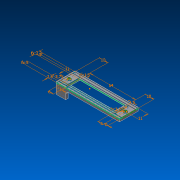
# Autodesk Inventor part: ethernet bracket
Saved by Autodesk Inventor 2015 (Build 190159000, 159)
## iProperties
Created: 2017-03-16
Part Number: ethernet bracket
Material: Generic
Document SubType Name: Modeling
Designer: ZigZagJoe
Density: 1 g/cm^3
Appearance: Default
Author: ZigZagJoe
Autodesk Inventor part; units mm, degrees
ref_plane "YZ Plane" through (0, 0, 0) normal (1, 0, 0) x (0, 1, 0)
ref_plane "XZ Plane" through (0, 0, 0) normal (0, 1, 0) x (-1, 0, 0)
ref_plane "XY Plane" through (0, 0, 0) normal (0, 0, 1) x (1, 0, 0)
sketch "Sketch1" plane through (0, 0, 0) normal (0, 0, 1) x (1, 0, 0)
  line L0 (-15.681, 3.6583) -> (38.319, 3.6583)
  line L1 (38.319, 3.6583) -> (38.319, -8.3417)
  line L2 (38.319, -8.3417) -> (-15.681, -8.3417)
  line L3 (-15.681, -8.3417) -> (-15.681, 3.6583)
  line L4 (48.319, 8.6583) -> (-25.681, 8.6583)
  line L5 (-25.681, 8.6583) -> (-25.681, -13.3417)
  line L6 (-25.681, -13.3417) -> (48.319, -13.3417)
  line L7 (48.319, -13.3417) -> (48.319, 8.6583)
  line L8 (-25.681, 5.8583) -> (48.319, 5.8583)
  line L9 (-25.681, -10.5417) -> (-25.681, -13.3417)
  line L10 (-25.681, -10.5417) -> (-14.681, -10.5417)
  line L11 (-14.681, -13.3417) -> (-25.681, -13.3417)
  line L12 (-25.681, -13.3417) -> (-25.681, -10.5417)
  line L13 (-14.681, -10.5417) -> (-14.681, -13.3417)
  line L14 (-14.681, -10.5417) -> (48.319, -10.5417)
  point P0 (0, 0)
  dimension "d0" = 54
  dimension "d1" = 12
  dimension "d4" = 5
  dimension "d5" = 5
  dimension "d7" = 2.2
  dimension "d62" = 10
  dimension "d65" = 10
  dimension "d66" = 0
  dimension "d69" = 1
  dimension "d70" = 2.8
  constraints: 31 end point, 6 point on line, 5 horizontal, 5 parallel, 2 perpendicular, 1 vertical
  measures "d0" distance of L1.end L2.end
  measures "d1" distance of L0.end L1.end
  measures "d4" distance between parallel lines of L4 L0
  measures "d5" distance between parallel lines of L2 L6
  measures "d7" distance between parallel lines of L8 L0
  measures "d62" distance between parallel lines of L3 L5
  measures "d65" distance between parallel lines of L7 L1
  measures "d66" distance of L6.end point (48.319, -13.342)
  measures "d69" distance between parallel lines of L13 L3
  measures "d70" distance between parallel lines of L11 L10
extrude "Face" add sketch "Sketch1" along normal blind 1
extrude "Walls" add sketch "Sketch1" against normal blind 3 contours L7 L8 L5 L4 | L7 L6 L13 L14 | L10 L13 L6 L5
extrude "Screw Support" add sketch "Sketch1" against normal blind 12 contours L10 L13 L6 L5
fillet "Fillet3" radius 0.5 1 edges at (11.319, 5.8583, 0)
sketch "Sketch2" plane through (-25.681, 5.8583, -3) normal (0, -1, 0) x (1, 0, 0)
  line L0 (56.5, 0.5) -> (53, 0.5)
  line L1 (53, 0.5) -> (53, 2)
  line L2 (53, 2) -> (56.5, 2)
  line L3 (56.5, 2) -> (56.5, 0.5)
  line L4 (21, 0.5) -> (17.5, 0.5)
  line L5 (17.5, 0.5) -> (17.5, 2)
  line L6 (17.5, 2) -> (21, 2)
  line L7 (21, 2) -> (21, 0.5)
  line L8 (74, 2.5) -> (74, 0) projected
  line L9 (0, 2.5) -> (0, 0) projected
  line L10 (64, 3) -> (64, 4) projected
  line L11 (10, 3) -> (10, 4) projected
  line L12 (64, 3) -> (10, 3) projected
  point P0 (25.681, 3)
  point P1 (0, 4.5)
  dimension "d26" = 3.5
  dimension "d27" = 3.5
  dimension "d29" = 1.5
  dimension "d53" = 7.5
  dimension "d54" = 7.5
  dimension "d78" = 2.5
  constraints: 16 end point, 4 parallel, 2 horizontal, 2 perpendicular, 2 point on line
  measures "d26" distance between parallel lines of L3 L1
  measures "d27" distance of L4.start L4.end
  measures "d29" distance of L0.end L1.end
  measures "d53" distance from line of L2.end L10
  measures "d54" distance from line of L4.end L11
  measures "d78" distance between parallel lines of L4 L12
extrude "Notches" cut sketch "Sketch2" against normal blind 0.8
fillet "Fillet4" radius 0.8 2 edges at (29.069, 6.6583, -1) (-6.431, 6.6583, -1)
sketch "Sketch3" plane through (0, 0, 0) normal (0, 0, -1) x (-1, 0, 0)
  circle A0 centre (-44.319, -2.3417) radius 1.875
  circle A1 centre (21.681, -2.3417) radius 1.875
  line L0 (-48.319, -10.5417) -> (-48.319, 5.3583) projected
  line L1 (25.681, 5.3583) -> (25.681, -10.5417) projected
  line L2 (-38.319, -8.3417) -> (-38.319, 3.6583) projected
  line L3 (15.681, 3.6583) -> (15.681, -8.3417) projected
  line L4 (25.681, 8.6583) -> (-48.319, 8.6583) projected
  line L5 (25.681, 5.8583) -> (-48.319, 5.8583) projected
  line L6 (-39.819, 5.8583) -> (-48.319, 5.8583)
  line L7 (-48.319, 5.8583) -> (-48.319, -10.5417)
  line L8 (-48.319, -10.5417) -> (-39.819, -10.5417)
  line L9 (-39.819, -10.5417) -> (-39.819, 5.8583)
  line L10 (17.181, 5.8583) -> (25.681, 5.8583)
  line L11 (25.681, 5.8583) -> (25.681, -10.5417)
  line L12 (25.681, -10.5417) -> (17.181, -10.5417)
  line L13 (17.181, -10.5417) -> (17.181, 5.8583)
  line L14 (25.681, -10.5417) -> (15.681, -10.5417)
  line L15 (15.681, -10.5417) -> (15.681, -8.3417)
  line L16 (15.681, -8.3417) -> (25.681, -8.3417)
  line L17 (25.681, -8.3417) -> (25.681, -10.5417)
  point P0 (0, 0)
  dimension "d37" = 3.75
  dimension "d38" = 3.75
  dimension "d60" = 6
  dimension "d61" = 6
  dimension "d71" = 11
  dimension "d72" = 11
  dimension "d74" = 1.5
  dimension "d75" = 1.5
  constraints: 24 end point, 6 parallel, 3 horizontal, 3 perpendicular, 2 centre point, 2 point on line
  measures "d37" diameter of A0
  measures "d38" diameter of A1
  measures "d60" distance from line of L2 A0.centre
  measures "d61" distance from line of L3 A1.centre
  measures "d71" distance from line of L4 A0.centre
  measures "d72" distance from line of L4 A1.centre
  measures "d74" distance between parallel lines of L2 L9
  measures "d75" distance between parallel lines of L3 L13
extrude "Mounting holes" add sketch "Sketch3" along normal blind 3 contours L0 L7 L5 L9 L8 | L1 L16 L13 L5 L11 | L1 L12 L13 L16
extrude "Extrusion6" cut sketch "Sketch3" against normal blind 5 contours A0 | A1
fillet "Fillet9" radius 0.8 8 edges at (39.819, -2.5917, 0) (39.819, 5.7118, -0.1464) (39.819, 5.8583, -1.75) (39.819, -10.5417, -1.5) (-17.181, 5.7118, -0.1464) (-17.181, 5.8583, -1.75) (-17.181, -10.5417, -1.5) (-17.181, -2.5917, 0)
fillet "Fillet10" radius 3 1 edges at (-14.681, -11.9417, -3)
extrude "Extrusion7" cut sketch "Sketch3" along normal blind 5 contours L1 L12 L13 L16 | L13 L14 L15 L16
fillet "Fillet12" radius 1 5 edges at (39.5847, -10.3074, -0.2343) (-21.031, -10.5417, 0) (-16.031, -10.5417, 0) (11.669, -10.5417, 0) (-21.031, -8.3417, 0)
extrude "Extrusion8" add sketch "Sketch3" along normal blind 1 contours L1 L12 L13 L16 | L13 L14 L15 L16
fillet "Fillet13" radius 1 2 edges at (-21.431, -8.3417, -1) (-20.681, -10.5417, -1)
equation "\"d5\" = d4"
equation "\"d7\" = d8"
equation "\"d26\" = d27"
equation "\"d54\" = d53"
equation "\"d37\" = d38"
equation "\"d75\" = d74"
equation "\"d8\" = 2.2"
body "Solid1"
